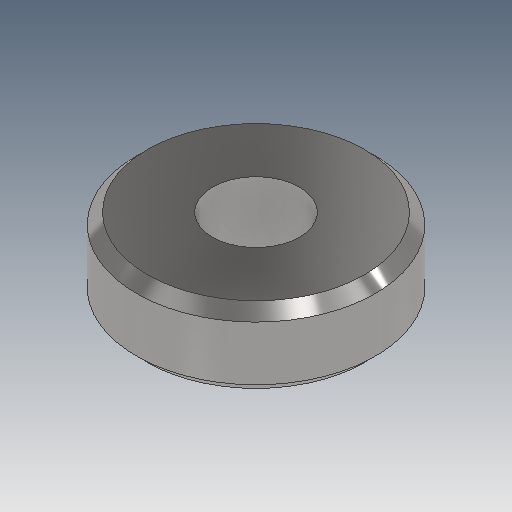
# Autodesk Inventor part: rolamento
Saved by Autodesk Inventor 2026.1 (Build 301233020, 233B)
## iProperties
Created: 2025-10-10
Part Number: rolamento
Material: Genérico
Document SubType Name: Modeling
Designer: Emmanuel Ribeiro
Density: 1 g/cm^3
Appearance: Padrão
Author: Emmanuel Ribeiro
Autodesk Inventor part; units mm, degrees
ref_plane "YZ Plane" through (0, 0, 0) normal (1, 0, 0) x (0, 1, 0)
ref_plane "XZ Plane" through (0, 0, 0) normal (0, 1, 0) x (-1, 0, 0)
ref_plane "XY Plane" through (0, 0, 0) normal (0, 0, 1) x (1, 0, 0)
sketch "Esboço1" plane through (0, 0, 0) normal (0, 1, 0) x (-1, 0, 0)
  circle A0 centre (0, 0) radius 11
  circle A1 centre (0, 0) radius 4
  dimension "d0" = 22
  dimension "d1" = 8
  constraints: 2 centre point, 2 coincident
  measures "d0" diameter of A0
  measures "d1" diameter of A1
extrude "Extrusão1" add sketch "Esboço1" along normal blind 7
chamfer "Chanfro1" distance 1 angle 45 2 edges at (11, 7, 0) (11, 0, 0)
